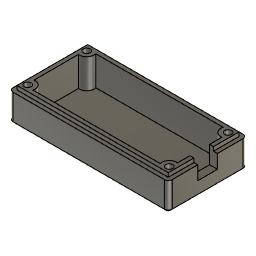
MG996R_Assembly v5 (Autodesk Fusion 360 archive; units mm, degrees)
design "MG996R_Shell_Bottom"
Autodesk Fusion 360 part; units mm, degrees
(part 1 of 2)
sketch "Sketch1" plane through (0, 0, 0) normal (0, 0, 1) x (1, 0, 0)
  line L0 (20.25, 10) -> (-20.25, 10)
  line L1 (-20.25, 10) -> (-20.25, -10)
  line L2 (-20.25, -10) -> (20.25, -10)
  line L3 (20.25, -10) -> (20.25, 10)
  line L4 (20.25, 10) -> (-20.25, -10) construction
  line L5 (-20.25, 10) -> (20.25, -10) construction
  dimension "d1" = 40.5
  dimension "d2" = 20
  constraint horizontal L0
  constraint perpendicular L0 L1
  constraint parallel L0 L2
  constraint parallel L1 L3
  constraint coincident L4 origin
  constraint coincident L5 origin
  measures "d1" distance of L0.start L0.end
  measures "d2" distance of L0.start L2.end
extrude "Extrude1" add sketch "Sketch1" along normal blind 8.53
sketch "Sketch2" plane through (0, 0, 8.53) normal (0, 0, 1) x (-1, 0, 0)
  line L0 (-20.25, 10) -> (-20.25, -10)
  line L1 (-20.25, -10) -> (20.25, -10)
  line L2 (20.25, -10) -> (20.25, 10)
  line L3 (20.25, 10) -> (-20.25, 10)
  line L4 (-18, -7.5) -> (18, -7.5) construction
  line L5 (18, -7.5) -> (18, 7.5) construction
  line L6 (18, 7.5) -> (-18, 7.5) construction
  line L7 (-18, 7.5) -> (-18, -7.5) construction
  line L8 (-18, -7.5) -> (18, 7.5) construction
  line L9 (18, -7.5) -> (-18, 7.5) construction
  circle A0 centre (-18, -7.5) radius 0.875
  circle A1 centre (-18, 7.5) radius 0.875
  circle A2 centre (18, 7.5) radius 0.875
  circle A3 centre (18, -7.5) radius 0.875
  dimension "d6" = 15
  dimension "d7" = 36
  dimension "d8" = 1.75
  constraint horizontal L4
  constraint perpendicular L4 L5
  constraint parallel L4 L6
  constraint parallel L5 L7
  constraint coincident L8 origin
  constraint coincident L9 origin
  constraint coincident L4.start L7.end
  constraint coincident L6.end L7.start
  constraint coincident L5.end L6.start
  constraint coincident L4.end L5.start
  constraint equal A2 A3
  constraint equal A0 A2
  constraint equal A0 A1
  measures "d6" distance of L4.end L5.end
  measures "d7" distance of L4.start L4.end
  measures "d8" diameter of A3
extrude "Extrude2" cut sketch "Sketch2" against normal blind 15 contours A0 | A1 | A2 | A3
sketch "Sketch3" plane through (0, 0, 8.53) normal (0, 0, 1) x (-1, 0, 0)
  circle A0 centre (-18, -7.5) radius 0.875
  circle A1 centre (-18, 7.5) radius 0.875
  circle A2 centre (18, -7.5) radius 0.875
  circle A3 centre (18, 7.5) radius 0.875
  line L0 (-20.25, 10) -> (-20.25, -10)
  line L1 (-20.25, -10) -> (20.25, -10)
  line L2 (20.25, -10) -> (20.25, 10)
  line L3 (20.25, 10) -> (-20.25, 10)
  line L4 (-18.25, -8) -> (18.25, -8)
  line L5 (18.25, -8) -> (18.25, 8)
  line L6 (18.25, 8) -> (-18.25, 8)
  line L7 (-18.25, 8) -> (-18.25, -8)
  line L8 (-18.25, -8) -> (18.25, 8) construction
  line L9 (18.25, -8) -> (-18.25, 8) construction
  circle A4 centre (-18, -7.5) radius 1.875
  circle A5 centre (-18, 7.5) radius 1.875
  circle A6 centre (18, 7.5) radius 1.875
  circle A7 centre (18, -7.5) radius 1.875
  dimension "d11" = 2
  dimension "d13" = 2
  dimension "d14" = 3.75
  constraint horizontal L4
  constraint perpendicular L4 L5
  constraint parallel L4 L6
  constraint parallel L5 L7
  constraint coincident L8 origin
  constraint coincident L9 origin
  constraint concentric A0 A4
  constraint concentric A1 A5
  constraint concentric A3 A6
  constraint concentric A2 A7
  constraint equal A6 A7
  constraint equal A5 A6
  constraint equal A4 A5
  measures "d11" distance of L1 L4
  measures "d13" distance of L0 L7
  measures "d14" diameter of A7
extrude "Extrude3" cut sketch "Sketch3" against normal blind 7.5 contours L4 L5 L6 L7 A4 A5 A6 A7
sketch "Sketch4" plane through (20.25, 0, 0) normal (1, 0, 0) x (0, 1, 0)
  line L0 (-10, 0) -> (10, 0)
  line L1 (10, 0) -> (10, 8.53)
  line L2 (10, 8.53) -> (-10, 8.53)
  line L3 (-10, 8.53) -> (-10, 0)
  line L4 (-2.5, 8.53) -> (2.5, 8.53)
  line L5 (2.5, 8.53) -> (2.5, 4.03)
  line L6 (2.5, 4.03) -> (-2.5, 4.03)
  line L7 (-2.5, 4.03) -> (-2.5, 8.53)
  dimension "d17" = 5
  dimension "d18" = 4.5
  dimension "d19" = 2.5
  constraint horizontal L4
  constraint vertical L5
  constraint horizontal L6
  constraint vertical L7
  constraint coincident L2 L4.start
  measures "d17" distance of L4.start L4.end
  measures "d18" distance of L4.start L6.end
  measures "d19" distance of origin L7
extrude "Extrude4" cut sketch "Sketch4" against normal blind 3 contours L2 L4 L5 L6 L7
sketch "Sketch5" plane through (0, 0, 8.53) normal (0, 0, 1) x (-1, 0, 0)
  line L0 (-20.25, 2.5) -> (-18.25, 2.5)
  line L1 (-18.25, 2.5) -> (-18.25, 5.6417)
  arc A0 (-18.25, 5.6417) -> (-16.1929, 8) centre (-18, 7.5) ccw
  line L2 (-16.1929, 8) -> (16.1929, 8)
  arc A1 (16.1929, 8) -> (18.25, 5.6417) centre (18, 7.5) ccw
  line L3 (18.25, 5.6417) -> (18.25, -5.6417)
  arc A2 (18.25, -5.6417) -> (16.1929, -8) centre (18, -7.5) ccw
  line L4 (16.1929, -8) -> (-16.1929, -8)
  arc A3 (-16.1929, -8) -> (-18.25, -5.6417) centre (-18, -7.5) ccw
  line L5 (-18.25, -5.6417) -> (-18.25, -2.5)
  line L6 (-18.25, -2.5) -> (-20.25, -2.5)
  line L7 (-20.25, -2.5) -> (-20.25, -10)
  line L8 (-20.25, -10) -> (20.25, -10)
  line L9 (20.25, -10) -> (20.25, 10)
  line L10 (20.25, 10) -> (-20.25, 10)
  line L11 (-20.25, 10) -> (-20.25, 2.5)
  circle A4 centre (-18, -7.5) radius 0.875
  circle A5 centre (-18, 7.5) radius 0.875
  circle A6 centre (18, -7.5) radius 0.875
  circle A7 centre (18, 7.5) radius 0.875
  line L12 (19.25, -9) -> (-19.25, -9)
  line L13 (-19.25, -9) -> (-19.25, 9)
  line L14 (-19.25, 9) -> (19.25, 9)
  line L15 (19.25, 9) -> (19.25, -9)
  line L16 (19.25, -9) -> (-19.25, 9) construction
  line L17 (-19.25, -9) -> (19.25, 9) construction
  dimension "d22" = 1
  dimension "d23" = 1
  constraint horizontal L12
  constraint perpendicular L12 L13
  constraint parallel L12 L14
  constraint parallel L13 L15
  constraint coincident L16 origin
  constraint coincident L17 origin
  measures "d22" distance of L8 L12
  measures "d23" distance of L9 L15
extrude "Extrude5" cut sketch "Sketch5" against normal blind 1 contours L0 L6 L7 L8 L9 L10 L11 L12 L13 L14 L15
fillet "Fillet1" radius 1 4 edges at (-20.25, -10, 3.765) (-20.25, 10, 3.765) (20.25, -10, 3.765) (20.25, 10, 3.765)
chamfer "Chamfer1" distance 1 angle 45 8 edges at (0, 10, 0) (-19.9571, 9.7071, 0) (-20.25, 0, 0) (-19.9571, -9.7071, 0) (0, -10, 0) (19.9571, -9.7071, 0) (20.25, 0, 0) (19.9571, 9.7071, 0)
sketch "Sketch6" plane through (0, 0, 0) normal (0, 0, -1) x (1, 0, 0)
  circle A0 centre (-18, 7.5) radius 0.875
  circle A1 centre (-18, -7.5) radius 0.875
  circle A2 centre (18, 7.5) radius 0.875
  circle A3 centre (18, -7.5) radius 0.875
  line L0 (-19.25, -9) -> (19.25, -9)
  line L1 (19.25, -9) -> (19.25, 9)
  line L2 (19.25, 9) -> (-19.25, 9)
  line L3 (-19.25, 9) -> (-19.25, -9)
  circle A4 centre (-19.25, 9) radius 5
  circle A5 centre (19.25, 9) radius 5
  circle A6 centre (19.25, -9) radius 5
  circle A7 centre (-19.25, -9) radius 5
  dimension "d29" = 10
  constraint equal A4 A7
  constraint equal A4 A5
  constraint equal A5 A6
  constraint coincident L2.end L3.start
  constraint coincident L0.start L3.end
  constraint coincident L1.end L2.start
  constraint coincident L0.end L1.start
  measures "d29" diameter of A4
extrude "Extrude6" cut sketch "Sketch6" against normal blind 0.5 contours L0 L3 A7 | L0 L3 A7 | L0 L1 A6 | L0 L1 A6 | L2 L3 A4 | L2 L3 A4 | L1 L2 A5 | L1 L2 A5

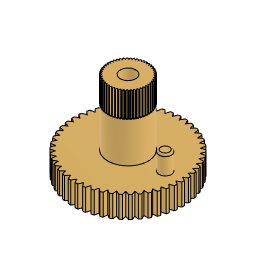
design "MG996R_Gear_4"
Autodesk Fusion 360 part; units mm, degrees
sketch "Sketch1" plane through (0, 0, 0) normal (0, 0, 1) x (1, 0, 0)
  circle A0 centre (0, 0) radius 8.9
  circle A1 centre (0, 0) radius 3.25
  dimension "d1" = 17.8
  dimension "d2" = 6.5
  constraint coincident A0.centre A1.centre
  measures "d1" diameter of A0
  measures "d2" diameter of A1
extrude "Extrude1" add sketch "Sketch1" along normal blind 3.5
sketch "Sketch2" plane through (0, 0, 0) normal (0, 0, -1) x (1, 0, 0)
  circle A0 centre (0, 0) radius 3.25
  circle A1 centre (0, 0) radius 8.9
  circle A2 centre (0, 0) radius 6
  circle A3 centre (0, 0) radius 5
  dimension "d5" = 12
  dimension "d6" = 10
  constraint coincident A0.centre A1.centre
  measures "d5" diameter of A2
  measures "d6" diameter of A3
extrude "Extrude2" add sketch "Sketch2" along normal blind 1 contours A2
extrude "Extrude3" add sketch "Sketch1" along normal blind 14 contours A1
sketch "Sketch4" plane through (0, 0, 14) normal (0, 0, 1) x (-1, 0, 0)
  circle A0 centre (0, 0) radius 3.25
  circle A1 centre (0, 0) radius 1.25
  dimension "d11" = 2.5
  constraint concentric A0 A1
  measures "d11" diameter of A1
extrude "Extrude4" cut sketch "Sketch4" against normal blind 37 contours A1
extrude "Extrude5" cut 1 faces at (3.7314, 0.2484, 0) along direction (0, 0, 1) blind 1.5
sketch "Sketch5" plane through (0, 0, 14) normal (0, 0, 1) x (-1, 0, 0)
  circle A0 centre (0, 0) radius 1.25
  circle A1 centre (0, 0) radius 3.25
  circle A2 centre (0, 0) radius 3.25
  line L0 (0.15, -3.2465) -> (0, -2.9867)
  line L1 (0, -2.9867) -> (-0.15, -3.2465)
  dimension "d16" = 0.3
  dimension "d17" = 0.3
  constraint concentric A0 A2
  constraint coincident A2 L0.start
  constraint coincident A2 L1.end
  constraint equal L0 L1
  constraint equal A1 A2
  constraint vertical A0.centre L0.end
  measures "d16" distance of L0.start L0.end
  measures "d17" distance of L0.start L1.end
extrude "Extrude6" cut sketch "Sketch5" against normal blind 4 contours A1 A2 L0 L1 picked at (0, -3.162)
pattern_circular "C-Pattern1" count 50 over 360 about axis through (0, 0, 14) along (0, 0, -1) of "Extrude6"
sketch "Sketch6" plane through (0, 0, 3.5) normal (0, 0, 1) x (-1, 0, 0)
  circle A0 centre (0, 0) radius 3.25
  circle A1 centre (0, 0) radius 8.9
  circle A2 centre (0, 0) radius 8.9
  line L0 (0.35, -8.8931) -> (0, -8.2869)
  line L1 (0, -8.2869) -> (-0.35, -8.8931)
  dimension "d22" = 0.7
  dimension "d23" = 0.7
  dimension "d24" = 0.7
  constraint coincident A0.centre A1.centre
  constraint coincident A2 L0.start
  constraint coincident A2 L1.end
  constraint equal A1 A2
  constraint vertical A0.centre L0.end
  measures "d22" distance of L0.start L0.end
  measures "d23" distance of L0.end L1.end
  measures "d24" horizontal distance of L0.start L1.end
extrude "Extrude7" cut sketch "Sketch6" against normal blind 6.5 contours A1 A2 L0 L1 picked at (0, -8.6951)
pattern_circular "C-Pattern2" count 50 over 360 about axis through (0, 0, 14) along (0, 0, -1) of "Extrude7"
sketch "Sketch7" plane through (0, 0, 3.5) normal (0, 0, 1) x (-1, 0, 0)
  line L0 (1.0386, -8.2216) -> (1.4618, -8.7791)
  arc A0 (1.4618, -8.7791) -> (1.8726, -8.7008) centre (0, 0) ccw
  line L1 (1.8726, -8.7008) -> (2.0609, -8.0265)
  line L2 (2.0609, -8.0265) -> (2.5506, -8.5267)
  arc A1 (2.5506, -8.5267) -> (2.9484, -8.3975) centre (0, 0) ccw
  line L3 (2.9484, -8.3975) -> (3.0506, -7.705)
  line L4 (3.0506, -7.705) -> (3.5992, -8.1398)
  arc A2 (3.5992, -8.1398) -> (3.9776, -7.9617) centre (0, 0) ccw
  line L5 (3.9776, -7.9617) -> (3.9922, -7.2619)
  line L6 (3.9922, -7.2619) -> (4.591, -7.6245)
  arc A3 (4.591, -7.6245) -> (4.9441, -7.4004) centre (0, 0) ccw
  line L7 (4.9441, -7.4004) -> (4.8709, -6.7042)
  line L8 (4.8709, -6.7042) -> (5.5104, -6.989)
  arc A4 (5.5104, -6.989) -> (5.8326, -6.7224) centre (0, 0) ccw
  line L9 (5.8326, -6.7224) -> (5.6728, -6.0409)
  line L10 (5.6728, -6.0409) -> (6.3429, -6.2432)
  arc A5 (6.3429, -6.2432) -> (6.6292, -5.9384) centre (0, 0) ccw
  line L11 (6.6292, -5.9384) -> (6.3852, -5.2823)
  line L12 (6.3852, -5.2823) -> (7.0754, -5.399)
  arc A6 (7.0754, -5.399) -> (7.3212, -5.0607) centre (0, 0) ccw
  line L13 (7.3212, -5.0607) -> (6.9969, -4.4403)
  line L14 (6.9969, -4.4403) -> (7.6962, -4.4697)
  arc A7 (7.6962, -4.4697) -> (7.8977, -4.1032) centre (0, 0) ccw
  line L15 (7.8977, -4.1032) -> (7.4982, -3.5284)
  line L16 (7.4982, -3.5284) -> (8.1958, -3.4698)
  arc A8 (8.1958, -3.4698) -> (8.3497, -3.081) centre (0, 0) ccw
  line L17 (8.3497, -3.081) -> (7.8813, -2.5608)
  line L18 (7.8813, -2.5608) -> (8.566, -2.4153)
  arc A9 (8.566, -2.4153) -> (8.67, -2.0102) centre (0, 0) ccw
  line L19 (8.67, -2.0102) -> (8.1401, -1.5528)
  line L20 (8.1401, -1.5528) -> (8.8012, -1.3226)
  arc A10 (8.8012, -1.3226) -> (8.8536, -0.9077) centre (0, 0) ccw
  line L21 (8.8536, -0.9077) -> (8.2705, -0.5203)
  line L22 (8.2705, -0.5203) -> (8.8975, -0.2091)
  arc A11 (8.8975, -0.2091) -> (8.8975, 0.2091) centre (0, 0) ccw
  line L23 (8.8975, 0.2091) -> (8.2705, 0.5203)
  line L24 (8.2705, 0.5203) -> (8.8536, 0.9077)
  arc A12 (8.8536, 0.9077) -> (8.8012, 1.3226) centre (0, 0) ccw
  line L25 (8.8012, 1.3226) -> (8.1401, 1.5528)
  line L26 (8.1401, 1.5528) -> (8.67, 2.0102)
  arc A13 (8.67, 2.0102) -> (8.566, 2.4153) centre (0, 0) ccw
  line L27 (8.566, 2.4153) -> (7.8813, 2.5608)
  line L28 (7.8813, 2.5608) -> (8.3497, 3.081)
  arc A14 (8.3497, 3.081) -> (8.1958, 3.4698) centre (0, 0) ccw
  line L29 (8.1958, 3.4698) -> (7.4982, 3.5284)
  line L30 (7.4982, 3.5284) -> (7.8977, 4.1032)
  arc A15 (7.8977, 4.1032) -> (7.6962, 4.4697) centre (0, 0) ccw
  line L31 (7.6962, 4.4697) -> (6.9969, 4.4403)
  line L32 (6.9969, 4.4403) -> (7.3212, 5.0607)
  arc A16 (7.3212, 5.0607) -> (7.0754, 5.399) centre (0, 0) ccw
  line L33 (7.0754, 5.399) -> (6.3852, 5.2823)
  line L34 (6.3852, 5.2823) -> (6.6292, 5.9384)
  arc A17 (6.6292, 5.9384) -> (6.3429, 6.2432) centre (0, 0) ccw
  line L35 (6.3429, 6.2432) -> (5.6728, 6.0409)
  line L36 (5.6728, 6.0409) -> (5.8326, 6.7224)
  arc A18 (5.8326, 6.7224) -> (5.5104, 6.989) centre (0, 0) ccw
  line L37 (5.5104, 6.989) -> (4.8709, 6.7042)
  line L38 (4.8709, 6.7042) -> (4.9441, 7.4004)
  arc A19 (4.9441, 7.4004) -> (4.591, 7.6245) centre (0, 0) ccw
  line L39 (4.591, 7.6245) -> (3.9922, 7.2619)
  line L40 (3.9922, 7.2619) -> (3.9776, 7.9617)
  arc A20 (3.9776, 7.9617) -> (3.5992, 8.1398) centre (0, 0) ccw
  line L41 (3.5992, 8.1398) -> (3.0506, 7.705)
  line L42 (3.0506, 7.705) -> (2.9484, 8.3975)
  arc A21 (2.9484, 8.3975) -> (2.5506, 8.5267) centre (0, 0) ccw
  line L43 (2.5506, 8.5267) -> (2.0609, 8.0265)
  line L44 (2.0609, 8.0265) -> (1.8726, 8.7008)
  arc A22 (1.8726, 8.7008) -> (1.4618, 8.7791) centre (0, 0) ccw
  line L45 (1.4618, 8.7791) -> (1.0386, 8.2216)
  line L46 (1.0386, 8.2216) -> (0.7674, 8.8669)
  arc A23 (0.7674, 8.8669) -> (0.35, 8.8931) centre (0, 0) ccw
  line L47 (0.35, 8.8931) -> (0, 8.2869)
  line L48 (0, 8.2869) -> (-0.35, 8.8931)
  arc A24 (-0.35, 8.8931) -> (-0.7674, 8.8669) centre (0, 0) ccw
  line L49 (-0.7674, 8.8669) -> (-1.0386, 8.2216)
  line L50 (-1.0386, 8.2216) -> (-1.4618, 8.7791)
  arc A25 (-1.4618, 8.7791) -> (-1.8726, 8.7008) centre (0, 0) ccw
  line L51 (-1.8726, 8.7008) -> (-2.0609, 8.0265)
  line L52 (-2.0609, 8.0265) -> (-2.5506, 8.5267)
  arc A26 (-2.5506, 8.5267) -> (-2.9484, 8.3975) centre (0, 0) ccw
  line L53 (-2.9484, 8.3975) -> (-3.0506, 7.705)
  line L54 (-3.0506, 7.705) -> (-3.5992, 8.1398)
  arc A27 (-3.5992, 8.1398) -> (-3.9776, 7.9617) centre (0, 0) ccw
  line L55 (-3.9776, 7.9617) -> (-3.9922, 7.2619)
  line L56 (-3.9922, 7.2619) -> (-4.591, 7.6245)
  arc A28 (-4.591, 7.6245) -> (-4.9441, 7.4004) centre (0, 0) ccw
  line L57 (-4.9441, 7.4004) -> (-4.8709, 6.7042)
  line L58 (-4.8709, 6.7042) -> (-5.5104, 6.989)
  arc A29 (-5.5104, 6.989) -> (-5.8326, 6.7224) centre (0, 0) ccw
  line L59 (-5.8326, 6.7224) -> (-5.6728, 6.0409)
  line L60 (-5.6728, 6.0409) -> (-6.3429, 6.2432)
  arc A30 (-6.3429, 6.2432) -> (-6.6292, 5.9384) centre (0, 0) ccw
  line L61 (-6.6292, 5.9384) -> (-6.3852, 5.2823)
  line L62 (-6.3852, 5.2823) -> (-7.0754, 5.399)
  arc A31 (-7.0754, 5.399) -> (-7.3212, 5.0607) centre (0, 0) ccw
  line L63 (-7.3212, 5.0607) -> (-6.9969, 4.4403)
  line L64 (-6.9969, 4.4403) -> (-7.6962, 4.4697)
  arc A32 (-7.6962, 4.4697) -> (-7.8977, 4.1032) centre (0, 0) ccw
  line L65 (-7.8977, 4.1032) -> (-7.4982, 3.5284)
  line L66 (-7.4982, 3.5284) -> (-8.1958, 3.4698)
  arc A33 (-8.1958, 3.4698) -> (-8.3497, 3.081) centre (0, 0) ccw
  line L67 (-8.3497, 3.081) -> (-7.8813, 2.5608)
  line L68 (-7.8813, 2.5608) -> (-8.566, 2.4153)
  arc A34 (-8.566, 2.4153) -> (-8.67, 2.0102) centre (0, 0) ccw
  line L69 (-8.67, 2.0102) -> (-8.1401, 1.5528)
  line L70 (-8.1401, 1.5528) -> (-8.8012, 1.3226)
  arc A35 (-8.8012, 1.3226) -> (-8.8536, 0.9077) centre (0, 0) ccw
  line L71 (-8.8536, 0.9077) -> (-8.2705, 0.5203)
  line L72 (-8.2705, 0.5203) -> (-8.8975, 0.2091)
  arc A36 (-8.8975, 0.2091) -> (-8.8975, -0.2091) centre (0, 0) ccw
  line L73 (-8.8975, -0.2091) -> (-8.2705, -0.5203)
  line L74 (-8.2705, -0.5203) -> (-8.8536, -0.9077)
  arc A37 (-8.8536, -0.9077) -> (-8.8012, -1.3226) centre (0, 0) ccw
  line L75 (-8.8012, -1.3226) -> (-8.1401, -1.5528)
  line L76 (-8.1401, -1.5528) -> (-8.67, -2.0102)
  arc A38 (-8.67, -2.0102) -> (-8.566, -2.4153) centre (0, 0) ccw
  line L77 (-8.566, -2.4153) -> (-7.8813, -2.5608)
  line L78 (-7.8813, -2.5608) -> (-8.3497, -3.081)
  arc A39 (-8.3497, -3.081) -> (-8.1958, -3.4698) centre (0, 0) ccw
  line L79 (-8.1958, -3.4698) -> (-7.4982, -3.5284)
  line L80 (-7.4982, -3.5284) -> (-7.8977, -4.1032)
  arc A40 (-7.8977, -4.1032) -> (-7.6962, -4.4697) centre (0, 0) ccw
  line L81 (-7.6962, -4.4697) -> (-6.9969, -4.4403)
  line L82 (-6.9969, -4.4403) -> (-7.3212, -5.0607)
  arc A41 (-7.3212, -5.0607) -> (-7.0754, -5.399) centre (0, 0) ccw
  line L83 (-7.0754, -5.399) -> (-6.3852, -5.2823)
  line L84 (-6.3852, -5.2823) -> (-6.6292, -5.9384)
  arc A42 (-6.6292, -5.9384) -> (-6.3429, -6.2432) centre (0, 0) ccw
  line L85 (-6.3429, -6.2432) -> (-5.6728, -6.0409)
  line L86 (-5.6728, -6.0409) -> (-5.8326, -6.7224)
  arc A43 (-5.8326, -6.7224) -> (-5.5104, -6.989) centre (0, 0) ccw
  line L87 (-5.5104, -6.989) -> (-4.8709, -6.7042)
  line L88 (-4.8709, -6.7042) -> (-4.9441, -7.4004)
  arc A44 (-4.9441, -7.4004) -> (-4.591, -7.6245) centre (0, 0) ccw
  line L89 (-4.591, -7.6245) -> (-3.9922, -7.2619)
  line L90 (-3.9922, -7.2619) -> (-3.9776, -7.9617)
  arc A45 (-3.9776, -7.9617) -> (-3.5992, -8.1398) centre (0, 0) ccw
  line L91 (-3.5992, -8.1398) -> (-3.0506, -7.705)
  line L92 (-3.0506, -7.705) -> (-2.9484, -8.3975)
  arc A46 (-2.9484, -8.3975) -> (-2.5506, -8.5267) centre (0, 0) ccw
  line L93 (-2.5506, -8.5267) -> (-2.0609, -8.0265)
  line L94 (-2.0609, -8.0265) -> (-1.8726, -8.7008)
  arc A47 (-1.8726, -8.7008) -> (-1.4618, -8.7791) centre (0, 0) ccw
  line L95 (-1.4618, -8.7791) -> (-1.0386, -8.2216)
  line L96 (-1.0386, -8.2216) -> (-0.7674, -8.8669)
  arc A48 (-0.7674, -8.8669) -> (-0.35, -8.8931) centre (0, 0) ccw
  line L97 (-0.35, -8.8931) -> (0, -8.2869)
  line L98 (0, -8.2869) -> (0.35, -8.8931)
  arc A49 (0.35, -8.8931) -> (0.7674, -8.8669) centre (0, 0) ccw
  line L99 (0.7674, -8.8669) -> (1.0386, -8.2216)
  circle A50 centre (0, 0) radius 3.25
  circle A51 centre (-6, 0) radius 1
  dimension "d29" = 2
  dimension "d30" = 6
  measures "d29" diameter of A51
  measures "d30" distance of A0.centre A51.centre
extrude "Extrude8" add sketch "Sketch7" along normal blind 3 contours A51
fillet "Fillet1" radius 0.3 1 edges at (6.9323, 0.3616, 6.5)
sketch "Sketch8" plane through (0, 0, 1.5) normal (0, 0, -1) x (1, 0, 0)
  circle A0 centre (0, 0) radius 1.25
  circle A1 centre (0, 0) radius 5
  line L0 (-1.5, -1) -> (1.5, -1)
  arc A2 (1.5, -1) -> (1.5, 1) centre (1.5, 0) ccw
  line L1 (1.5, 1) -> (-1.5, 1)
  arc A3 (-1.5, 1) -> (-1.5, -1) centre (-1.5, 0) ccw
  line L2 (-1.5, 0) -> (1.5, 0) construction
  dimension "d35" = 2
  dimension "d36" = 3
  constraint tangent L0 A2
  constraint tangent A2 L1
  constraint parallel L0 L1
  constraint tangent L1 A3
  constraint tangent L0 A3
  constraint horizontal L2
  constraint coincident A0.centre A1.centre
  constraint midpoint L2 A0.centre
  measures "d35" distance of L0 L1
  measures "d36" distance of A3.centre A2.centre
extrude "Extrude9" cut sketch "Sketch8" against normal blind 4 contours A0 L0 A2 L1 | A0 L0 L1 A3

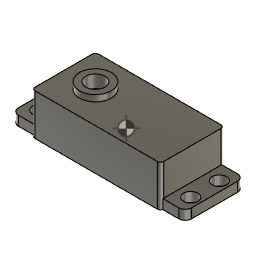
design "MG996R_Shell_Top"
Autodesk Fusion 360 part; units mm, degrees
sketch "Sketch1" plane through (0, 0, 0) normal (0, 0, 1) x (1, 0, 0)
  line L0 (-19.8608, 0) -> (46.1392, 0) construction
  line L1 (-17, -9.25) -> (-10, -9.25)
  line L2 (-10, -9.25) -> (-10, -10)
  line L3 (-10, -10) -> (30.5, -10)
  line L4 (30.5, -10) -> (30.5, -9.25)
  line L5 (30.5, -9.25) -> (37.5, -9.25)
  line L6 (37.5, -9.25) -> (37.5, 0)
  circle A0 centre (-13, -4.5) radius 2.25
  line L7 (-17, -9.25) -> (-17, 0)
  circle A1 centre (34.5, -4.5) radius 2.25
  line L8 (30.5, 10) -> (30.5, 9.25)
  line L9 (-10, 9.25) -> (-10, 10)
  line L10 (-17, 9.25) -> (-17, 0)
  line L11 (37.5, 9.25) -> (37.5, 0)
  line L12 (30.5, 9.25) -> (37.5, 9.25)
  circle A2 centre (-13, 4.5) radius 2.25
  line L13 (-10, 10) -> (30.5, 10)
  line L14 (-17, 9.25) -> (-10, 9.25)
  circle A3 centre (34.5, 4.5) radius 2.25
  point P0 (46.1392, 0)
  point P1 (-19.8608, 0)
  dimension "d1" = 4.5
  dimension "d2" = 10
  dimension "d3" = 4.5
  dimension "d4" = 47.5
  dimension "d5" = 7
  dimension "d6" = 7
  dimension "d7" = 4
  dimension "d8" = 4
  dimension "d9" = 4.5
  dimension "d10" = 4.5
  dimension "d11" = 10
  dimension "d12" = 10
  dimension "d13" = 9.25
  dimension "d14" = 9.25
  constraint horizontal L0
  constraint perpendicular L1 L2
  constraint perpendicular L3 L4
  constraint perpendicular L4 L5
  constraint coincident L0 L6.end
  constraint perpendicular L0 L6
  constraint coincident L0 L7.end
  constraint perpendicular L0 L7
  constraint coincident origin L0
  constraint symmetric P1 L0 L0.start
  constraint symmetric P0 L0 L0.end
  constraint symmetric L0 L1.start L10.start
  constraint symmetric L0 L1.end L9.start
  constraint symmetric L0 L2.end L9.end
  constraint symmetric L0 L3.end L8.start
  constraint symmetric L0 L4.end L8.end
  constraint symmetric L0 L5.end L11.start
  constraint symmetric L0 L6.end L11.end
  constraint symmetric L0 A0 A2
  constraint symmetric L0 L7.end L10.end
  constraint symmetric L0 A1 A3
  measures "d1" diameter of A1
  measures "d2" distance of L0 L3
  measures "d3" distance of L0 A1.centre
  measures "d4" horizontal distance of A0.centre A1.centre
  measures "d5" distance of L2 L7
  measures "d6" distance of L4 L6
  measures "d7" distance of L4 A1.centre
  measures "d8" distance of A0.centre L7
  measures "d9" diameter of A0
  measures "d10" distance of L0 A0.centre
  measures "d11" distance of origin L2
  measures "d12" distance of L0 L3
  measures "d13" distance of L0 L1
  measures "d14" distance of L0 L5
extrude "Extrude1" add sketch "Sketch1" along normal blind 13
sketch "Sketch3" plane through (0, -9.25, 0) normal (0, -1, 0) x (1, 0, 0)
  line L0 (30.5, 0) -> (37.5, 0)
  line L1 (37.5, 0) -> (37.5, 13)
  line L2 (37.5, 13) -> (30.5, 13)
  line L3 (30.5, 13) -> (30.5, 0)
  line L4 (37.5, 0) -> (30.5, 0)
  line L5 (30.5, 0) -> (30.5, 3)
  line L6 (30.5, 3) -> (37.5, 3)
  line L7 (37.5, 3) -> (37.5, 0)
  line L8 (-10, 0) -> (-17, 0)
  line L9 (-17, 0) -> (-17, 3)
  line L10 (-17, 3) -> (-10, 3)
  line L11 (-10, 3) -> (-10, 0)
  dimension "d21" = 3
  dimension "d22" = 3
  constraint horizontal L4
  constraint vertical L5
  constraint horizontal L6
  constraint vertical L7
  constraint coincident L3 L5.end
  constraint coincident L0.end L1.start
  constraint horizontal L8
  constraint vertical L9
  constraint horizontal L10
  constraint vertical L11
  measures "d21" distance of L8.start L10.end
  measures "d22" distance of L0.start L5.end
extrude "Extrude3" cut sketch "Sketch3" against normal blind 26 contours L1 L2 L3 L6
sketch "Sketch4" plane through (0, -9.25, 0) normal (0, -1, 0) x (1, 0, 0)
  line L0 (-17, 0) -> (-10, 0)
  line L1 (-10, 0) -> (-10, 13)
  line L2 (-10, 13) -> (-17, 13)
  line L3 (-17, 13) -> (-17, 0)
  line L4 (-17, 0) -> (-10, 0)
  line L5 (-10, 0) -> (-10, 3)
  line L6 (-10, 3) -> (-17, 3)
  line L7 (-17, 3) -> (-17, 0)
  dimension "d25" = 3
  constraint horizontal L4
  constraint vertical L5
  constraint horizontal L6
  constraint vertical L7
  constraint coincident L1 L5.end
  constraint coincident L0.start L3.end
  measures "d25" distance of L0.start L6.end
extrude "Extrude4" cut sketch "Sketch4" against normal blind 22 contours L1 L2 L3 L6
sketch "Sketch5" plane through (0, 0, 13) normal (0, 0, 1) x (-1, 0, 0)
  line L0 (10, -10) -> (10, 10)
  line L1 (10, 10) -> (-30.5, 10)
  line L2 (-30.5, 10) -> (-30.5, -10)
  line L3 (-30.5, -10) -> (10, -10)
  circle A0 centre (0, 0) radius 3
  dimension "d28" = 6
  constraint coincident A0.centre origin
  measures "d28" diameter of A0
extrude "Extrude5" cut sketch "Sketch5" against normal blind 21 contours A0
sketch "Sketch6" plane through (0, 0, 0) normal (0, 0, -1) x (-1, 0, 0)
  circle A0 centre (0, 0) radius 3
  line L0 (10, -10) -> (10, 10)
  line L1 (10, 10) -> (-33, 10)
  line L2 (-33, 10) -> (-33, -10)
  line L3 (-33, -10) -> (10, -10)
  circle A1 centre (-11, 0) radius 0.75
  circle A2 centre (-20.5, 0) radius 0.75
  circle A3 centre (0, 0) radius 3
  circle A4 centre (-34.5, 4.5) radius 2.25
  circle A5 centre (13, -4.5) radius 2.25
  circle A6 centre (-34.5, -4.5) radius 2.25
  circle A7 centre (13, 4.5) radius 2.25
  line L4 (10, -9.25) -> (17, -9.25)
  line L5 (17, -9.25) -> (17, 9.25)
  line L6 (17, 9.25) -> (10, 9.25)
  line L7 (10, 9.25) -> (10, 10)
  line L8 (10, 10) -> (-30.5, 10)
  line L9 (-30.5, 10) -> (-30.5, 9.25)
  line L10 (-30.5, 9.25) -> (-37.5, 9.25)
  line L11 (-37.5, 9.25) -> (-37.5, -9.25)
  line L12 (-37.5, -9.25) -> (-30.5, -9.25)
  line L13 (-30.5, -9.25) -> (-30.5, -10)
  line L14 (-30.5, -10) -> (10, -10)
  line L15 (10, -10) -> (10, -9.25)
  dimension "d31" = 1.5
  dimension "d32" = 1.5
  dimension "d33" = 11
  dimension "d34" = 9.5
  measures "d31" diameter of A1
  measures "d32" diameter of A2
  measures "d33" distance of A0.centre A1.centre
  measures "d34" distance of A1.centre A2.centre
extrude "Extrude6" cut sketch "Sketch6" against normal blind 12 contours A1 | A2
sketch "Sketch7" plane through (0, 0, 0) normal (0, 0, -1) x (1, 0, 0)
  circle A0 centre (11, 0) radius 0.75
  circle A1 centre (20.5, 0) radius 0.75
  circle A2 centre (0, 0) radius 3
  circle A3 centre (34.5, -4.5) radius 2.25
  circle A4 centre (-13, 4.5) radius 2.25
  circle A5 centre (34.5, 4.5) radius 2.25
  circle A6 centre (-13, -4.5) radius 2.25
  line L0 (-10, 9.25) -> (-17, 9.25)
  line L1 (-17, 9.25) -> (-17, -9.25)
  line L2 (-17, -9.25) -> (-10, -9.25)
  line L3 (-10, -9.25) -> (-10, -10)
  line L4 (-10, -10) -> (30.5, -10)
  line L5 (30.5, -10) -> (30.5, -9.25)
  line L6 (30.5, -9.25) -> (37.5, -9.25)
  line L7 (37.5, -9.25) -> (37.5, 9.25)
  line L8 (37.5, 9.25) -> (30.5, 9.25)
  line L9 (30.5, 9.25) -> (30.5, 10)
  line L10 (30.5, 10) -> (-10, 10)
  line L11 (-10, 10) -> (-10, 9.25)
  line L12 (29.5, 9) -> (-9, 9)
  line L13 (-9, 9) -> (-9, -9)
  line L14 (-9, -9) -> (29.5, -9)
  line L15 (29.5, -9) -> (29.5, 9)
  line L16 (29.5, 9) -> (-9, -9) construction
  line L17 (-9, 9) -> (29.5, -9) construction
  point P0 (10.25, 0)
  dimension "d37" = 1
  dimension "d38" = 1
  dimension "d39" = 1
  dimension "d40" = 1
  constraint horizontal L12
  constraint perpendicular L12 L13
  constraint parallel L12 L14
  constraint parallel L13 L15
  constraint coincident L16 P0
  constraint coincident L17 P0
  measures "d37" distance of L10 L12
  measures "d38" distance of L4 L14
  measures "d39" distance of L5 L15
  measures "d40" distance of L11 L13
extrude "Extrude7" cut sketch "Sketch7" against normal blind 12 contours L12 L13 L14 L15
sketch "Sketch8" plane through (0, 0, 12) normal (0, 0, -1) x (1, 0, 0)
  circle A0 centre (0, 0) radius 3
  line L0 (29.5, -9) -> (29.5, 9)
  line L1 (29.5, 9) -> (-9, 9)
  line L2 (-9, 9) -> (-9, -9)
  line L3 (-9, -9) -> (29.5, -9)
  circle A1 centre (11, 0) radius 0.75
  circle A2 centre (20.5, 0) radius 0.75
  circle A3 centre (11, 0) radius 1.75
  circle A4 centre (20.5, 0) radius 1.75
  dimension "d43" = 1.5
  dimension "d44" = 1.5
  dimension "d45" = 9.5
  dimension "d46" = 11
  dimension "d47" = 3.5
  dimension "d48" = 3.5
  constraint concentric A1 A3
  constraint concentric A2 A4
  measures "d43" diameter of A1
  measures "d44" diameter of A2
  measures "d45" distance of A1.centre A2.centre
  measures "d46" distance of A0.centre A1.centre
  measures "d47" diameter of A3
  measures "d48" diameter of A4
extrude "Extrude8" add sketch "Sketch8" along normal blind 1 contours A3 | A4
sketch "Sketch9" plane through (0, 0, 12) normal (0, 0, -1) x (1, 0, 0)
  circle A0 centre (11, 0) radius 1.75
  circle A1 centre (0, 0) radius 3
  line L0 (29.5, -9) -> (29.5, 9)
  line L1 (29.5, 9) -> (-9, 9)
  line L2 (-9, 9) -> (-9, -9)
  line L3 (-9, -9) -> (29.5, -9)
  circle A2 centre (20.5, 0) radius 1.75
  circle A3 centre (0, 0) radius 3
  circle A4 centre (0, 0) radius 5
  dimension "d51" = 2
  constraint concentric A1 A3
  constraint concentric A3 A4
  measures "d51" distance of A3 A4
extrude "Extrude9" add sketch "Sketch9" along normal blind 1 contours A4
sketch "Sketch10" plane through (0, 0, 13) normal (0, 0, 1) x (-1, 0, 0)
  circle A0 centre (0, 0) radius 3
  line L0 (10, -10) -> (10, 10)
  line L1 (10, 10) -> (-30.5, 10)
  line L2 (-30.5, 10) -> (-30.5, -10)
  line L3 (-30.5, -10) -> (10, -10)
  circle A1 centre (0, 0) radius 3
  circle A2 centre (0, 0) radius 5
  dimension "d54" = 2
  constraint concentric A0 A1
  constraint concentric A1 A2
  measures "d54" distance of A1 A2
extrude "Extrude10" add sketch "Sketch10" along normal blind 2 contours A2
fillet "Fillet1" radius 1 4 edges at (30.5, -10, 6.5) (30.5, 10, 6.5) (-10, -10, 6.5) (-10, 10, 6.5)
fillet "Fillet2" radius 2 4 edges at (37.5, -9.25, 1.5) (37.5, 9.25, 1.5) (-17, -9.25, 1.5) (-17, 9.25, 1.5)
sketch "Sketch11" plane through (0, 0, 12) normal (0, 0, -1) x (1, 0, 0)
  circle A0 centre (0, 0) radius 5 construction
  circle A1 centre (11, 0) radius 1.75 construction
  line L0 (29.5, -9) -> (29.5, 9) construction
  line L1 (29.5, 9) -> (-9, 9) construction
  line L2 (-9, 9) -> (-9, -9) construction
  line L3 (-9, -9) -> (29.5, -9) construction
  circle A2 centre (20.5, 0) radius 1.75 construction
  line L4 (28.25, -7.5) -> (-7.75, -7.5) construction
  line L5 (-7.75, -7.5) -> (-7.75, 7.5) construction
  line L6 (-7.75, 7.5) -> (28.25, 7.5) construction
  line L7 (28.25, 7.5) -> (28.25, -7.5) construction
  circle A3 centre (-7.75, 7.5) radius 0.875
  circle A4 centre (-7.75, -7.5) radius 0.875
  circle A5 centre (28.25, 7.5) radius 0.875
  circle A6 centre (28.25, -7.5) radius 0.875
  circle A7 centre (28.25, 7.5) radius 1.875
  circle A8 centre (28.25, -7.5) radius 1.875
  circle A9 centre (-7.75, -7.5) radius 1.875
  circle A10 centre (-7.75, 7.5) radius 1.875
  line L8 (-9, 10) -> (29.5, 10)
  line L9 (-9, -10) -> (29.5, -10)
  dimension "d63" = 1.25
  dimension "d66" = 1.75
  dimension "d67" = 1
  dimension "d70" = 36
  dimension "d71" = 15
  dimension "d73" = 2.5
  dimension "d74" = 2.5
  dimension "d75" = 1.25
  dimension "d76" = 1.25
  constraint horizontal L4
  constraint vertical L5
  constraint horizontal L6
  constraint vertical L7
  constraint coincident L5.end L6.start
  constraint coincident L4.end L5.start
  constraint coincident L6.end L7.start
  constraint coincident L4.start L7.end
  constraint equal A5 A6
  constraint equal A3 A6
  constraint equal A3 A4
  constraint concentric A6 A8
  constraint concentric A4 A9
  constraint concentric A3 A10
  constraint equal A9 A10
  constraint equal A8 A9
  constraint equal A7 A8
  measures "d63" distance of L2 L5
  measures "d66" diameter of A5
  measures "d67" distance of A5 A7
  measures "d70" distance of L5.end L6.end
  measures "d71" distance of L4.start L6.end
  measures "d73" distance of L6 L8
  measures "d74" distance of L4 L9
  measures "d75" distance of L2 L5
  measures "d76" distance of L0 L7
extrude "Extrude11" add sketch "Sketch11" along normal blind 12
equation "d13 = ( 18.5 / 2 ) * 1 mm"
equation "d14 = ( 18.5 / 2 ) * 1 mm"

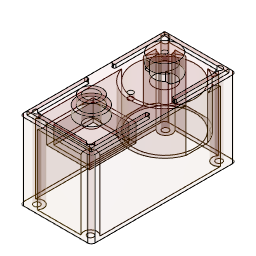
design "MG996R_Shell_Middle"
Autodesk Fusion 360 part; units mm, degrees
sketch "Sketch1" plane through (0, 0, 0) normal (0, 0, 1) x (1, 0, 0)
  line L0 (10, 20.25) -> (-10, 20.25)
  line L1 (-10, 20.25) -> (-10, -20.25)
  line L2 (-10, -20.25) -> (10, -20.25)
  line L3 (10, -20.25) -> (10, 20.25)
  line L4 (10, 20.25) -> (-10, -20.25) construction
  line L5 (-10, 20.25) -> (10, -20.25) construction
  dimension "d1" = 20
  dimension "d2" = 40.5
  constraint horizontal L0
  constraint perpendicular L0 L1
  constraint parallel L0 L2
  constraint parallel L1 L3
  constraint coincident L4 origin
  constraint coincident L5 origin
  measures "d1" distance of L0.start L0.end
  measures "d2" distance of L0.end L1.end
extrude "Extrude1" add sketch "Sketch1" along normal blind 21.5
sketch "Sketch2" plane through (0, 0, 21.5) normal (0, 0, 1) x (-1, 0, 0)
  line L0 (-10, 20.25) -> (-10, -20.25)
  line L1 (-10, -20.25) -> (10, -20.25)
  line L2 (10, -20.25) -> (10, 20.25)
  line L3 (10, 20.25) -> (-10, 20.25)
  line L4 (-8, -18.25) -> (8, -18.25)
  line L5 (8, -18.25) -> (8, 18.25)
  line L6 (8, 18.25) -> (-8, 18.25)
  line L7 (-8, 18.25) -> (-8, -18.25)
  line L8 (-8, -18.25) -> (8, 18.25) construction
  line L9 (8, -18.25) -> (-8, 18.25) construction
  line L10 (-9, -19.25) -> (9, -19.25)
  line L11 (9, -19.25) -> (9, 19.25)
  line L12 (9, 19.25) -> (-9, 19.25)
  line L13 (-9, 19.25) -> (-9, -19.25)
  line L14 (-9, -19.25) -> (9, 19.25) construction
  line L15 (9, -19.25) -> (-9, 19.25) construction
  dimension "d5" = 1
  dimension "d6" = 1
  dimension "d7" = 1
  dimension "d8" = 1
  constraint horizontal L4
  constraint perpendicular L4 L5
  constraint parallel L4 L6
  constraint parallel L5 L7
  constraint coincident L8 origin
  constraint coincident L9 origin
  constraint horizontal L10
  constraint perpendicular L10 L11
  constraint parallel L10 L12
  constraint parallel L11 L13
  constraint coincident L14 origin
  constraint coincident L15 origin
  measures "d5" distance of L4 L10
  measures "d6" distance of L7 L13
  measures "d7" distance of L0 L13
  measures "d8" distance of L1 L10
extrude "Extrude2" add sketch "Sketch2" along normal blind 1 contours L10 L11 L12 L13
sketch "Sketch3" plane through (0, 0, 21.5) normal (0, 0, 1) x (-1, 0, 0)
  line L0 (-8, -18.25) -> (8, -18.25)
  line L1 (8, -18.25) -> (8, 18.25)
  line L2 (8, 18.25) -> (-8, 18.25)
  line L3 (-8, 18.25) -> (-8, -18.25)
  circle A0 centre (0, 10.25) radius 2
  line L4 (10, 20.25) -> (-10, 20.25)
  circle A1 centre (0, -0.75) radius 0.75
  circle A2 centre (0, -10.25) radius 3
  line L5 (-10, -20.25) -> (10, -20.25)
  circle A3 centre (0, -10.25) radius 4
  circle A4 centre (0, 10.25) radius 4
  dimension "d11" = 4
  dimension "d12" = 10
  dimension "d13" = 11
  dimension "d14" = 9.5
  dimension "d16" = 10
  dimension "d17" = 1.5
  dimension "d18" = 6
  dimension "d19" = 8
  dimension "d20" = 8
  constraint vertical A1.centre A2.centre
  constraint vertical A0.centre A1.centre
  constraint vertical origin A1.centre
  constraint concentric A2 A3
  constraint concentric A0 A4
  measures "d11" diameter of A0
  measures "d12" distance of A0.centre L4
  measures "d13" vertical distance of A0.centre A1.centre
  measures "d14" distance of A1.centre A2.centre
  measures "d16" distance of A2.centre L5
  measures "d17" diameter of A1
  measures "d18" diameter of A2
  measures "d19" diameter of A4
  measures "d20" diameter of A3
extrude "Extrude3" add sketch "Sketch3" along normal blind 5 contours A3
extrude "Extrude4" add sketch "Sketch3" along normal blind 5 contours A4
sketch "Sketch4" plane through (0, 0, 26.5) normal (0, 0, 1) x (-1, 0, 0)
  circle A0 centre (0, 10.25) radius 2
  circle A1 centre (0, 10.25) radius 4
  circle A2 centre (0, 10.25) radius 3
  dimension "d25" = 6
  constraint concentric A0 A2
  measures "d25" diameter of A2
extrude "Extrude5" cut sketch "Sketch4" against normal blind 2.5 contours A1
extrude "Extrude6" cut sketch "Sketch3" against normal blind 1.5 contours A1
sketch "Sketch5" plane through (0, 0, 0) normal (0, 0, -1) x (1, 0, 0)
  line L0 (10, -20.25) -> (10, 20.25)
  line L1 (10, 20.25) -> (-10, 20.25)
  line L2 (-10, 20.25) -> (-10, -20.25)
  line L3 (-10, -20.25) -> (10, -20.25)
  line L4 (7.5, 18) -> (-7.5, 18) construction
  line L5 (-7.5, 18) -> (-7.5, -18) construction
  line L6 (-7.5, -18) -> (7.5, -18) construction
  line L7 (7.5, -18) -> (7.5, 18) construction
  line L8 (7.5, 18) -> (-7.5, -18) construction
  line L9 (-7.5, 18) -> (7.5, -18) construction
  circle A0 centre (-7.5, 18) radius 0.875
  circle A1 centre (7.5, 18) radius 0.875
  circle A2 centre (7.5, -18) radius 0.875
  circle A3 centre (-7.5, -18) radius 0.875
  dimension "d30" = 15
  dimension "d31" = 36
  dimension "d32" = 1.75
  constraint horizontal L4
  constraint perpendicular L4 L5
  constraint parallel L4 L6
  constraint parallel L5 L7
  constraint coincident L8 origin
  constraint coincident L9 origin
  constraint coincident L4.end L5.start
  constraint coincident L4.start L7.end
  constraint coincident L6.end L7.start
  constraint coincident L5.end L6.start
  constraint equal A0 A1
  constraint equal A1 A2
  constraint equal A2 A3
  measures "d30" distance of L4.start L4.end
  measures "d31" distance of L4.end L5.end
  measures "d32" diameter of A3
extrude "Extrude7" cut sketch "Sketch5" against normal blind 27 contours A0 | A1 | A2 | A3
sketch "Sketch6" plane through (0, 0, 0) normal (0, 0, -1) x (1, 0, 0)
  circle A0 centre (7.5, 18) radius 0.875
  circle A1 centre (7.5, -18) radius 0.875
  circle A2 centre (-7.5, 18) radius 0.875
  circle A3 centre (-7.5, -18) radius 0.875
  line L0 (10, -20.25) -> (10, 20.25)
  line L1 (10, 20.25) -> (-10, 20.25)
  line L2 (-10, 20.25) -> (-10, -20.25)
  line L3 (-10, -20.25) -> (10, -20.25)
  circle A4 centre (-7.5, 18) radius 1.875
  circle A5 centre (7.5, 18) radius 1.875
  circle A6 centre (7.5, -18) radius 1.875
  circle A7 centre (-7.5, -18) radius 1.875
  line L4 (9, 19.25) -> (-9, 19.25)
  line L5 (-9, 19.25) -> (-9, -19.25)
  line L6 (-9, -19.25) -> (9, -19.25)
  line L7 (9, -19.25) -> (9, 19.25)
  line L8 (9, 19.25) -> (-9, -19.25) construction
  line L9 (-9, 19.25) -> (9, -19.25) construction
  dimension "d35" = 3.75
  dimension "d36" = 1
  dimension "d37" = 1
  constraint concentric A2 A4
  constraint concentric A0 A5
  constraint concentric A1 A6
  constraint concentric A3 A7
  constraint equal A4 A7
  constraint equal A4 A5
  constraint equal A5 A6
  constraint horizontal L4
  constraint perpendicular L4 L5
  constraint parallel L4 L6
  constraint parallel L5 L7
  constraint coincident L8 origin
  constraint coincident L9 origin
  measures "d35" diameter of A7
  measures "d36" distance of L1 L4
  measures "d37" distance of L2 L5
extrude "Extrude8" cut sketch "Sketch6" against normal up to surface (19.5 mm away) contours A4 A5 A6 A7 L4 L5 L6 L7
extrude "Extrude9" cut 1 faces at (0.1483, -10.9, 21.5) along direction (0, 0, -1) blind 15
sketch "Sketch8" plane through (0, 0, 26.5) normal (0, 0, 1) x (-1, 0, 0)
  circle A0 centre (0, -10.25) radius 3
  circle A1 centre (0, -10.25) radius 4
  circle A2 centre (0, -10.25) radius 4
  constraint concentric A0 A2
extrude "Extrude10" add sketch "Sketch8" against normal blind 2.5 contours A0
ref_plane "WorkPlane1" through (0, 6.25, 22) normal (0, -1, 0) x (1, 0, 0)
sketch "Sketch10" plane through (0, 6.25, 22) normal (0, -1, 0) x (1, 0, 0)
  line L0 (-4, 2) -> (4, 2)
  line L1 (4, 2) -> (4, -0.5)
  line L2 (4, -0.5) -> (-4, -0.5)
  line L3 (-4, -0.5) -> (-4, 2)
  constraint horizontal L0
  constraint vertical L1
  constraint horizontal L2
  constraint vertical L3
extrude "Extrude11" cut sketch "Sketch10" against normal blind 2
sketch "Sketch11" plane through (0, 0, 26.5) normal (0, 0, 1) x (-1, 0, 0)
  circle A0 centre (0, -10.25) radius 4
  circle A1 centre (0, -10.25) radius 0.75
  dimension "d47" = 1.5
  constraint concentric A0 A1
  measures "d47" diameter of A1
extrude "Extrude12" cut sketch "Sketch11" against normal blind 1.5 contours A1
sketch "Sketch12" plane through (0, 0, 21.5) normal (0, 0, 1) x (-1, 0, 0)
  arc A0 (-3.4641, -8.25) -> (3.4641, -8.25) centre (0, -10.25) ccw
  line L0 (-3.4641, -8.25) -> (-2.2361, -8.25)
  arc A1 (-2.2361, -8.25) -> (2.2361, -8.25) centre (0, -10.25) ccw
  line L1 (2.2361, -8.25) -> (3.4641, -8.25)
  arc A2 (-8, 17.2819) -> (-6.6615, 18.25) centre (-7.5, 18) ccw
  line L2 (-8, 17.2819) -> (-8, -17.2819)
  arc A3 (-6.6615, -18.25) -> (-8, -17.2819) centre (-7.5, -18) ccw
  line L3 (-6.6615, -18.25) -> (6.6615, -18.25)
  arc A4 (8, -17.2819) -> (6.6615, -18.25) centre (7.5, -18) ccw
  line L4 (8, -17.2819) -> (8, 17.2819)
  arc A5 (6.6615, 18.25) -> (8, 17.2819) centre (7.5, 18) ccw
  line L5 (6.6615, 18.25) -> (-6.6615, 18.25)
  circle A6 centre (0, -0.75) radius 0.75
  circle A7 centre (0, 10.25) radius 4
  circle A8 centre (0, -10.25) radius 3
  dimension "d50" = 6
  constraint concentric A0 A8
  measures "d50" diameter of A8
extrude "Extrude13" cut sketch "Sketch12" against normal blind 4 contours A1 A8
sketch "Sketch13" plane through (0, 0, 21.5) normal (0, 0, 1) x (-1, 0, 0)
  arc A0 (2.2361, -8.25) -> (-2.2361, -8.25) centre (0, -10.25) ccw
  line L0 (2.2361, -8.25) -> (3.4641, -8.25)
  arc A1 (-3.4641, -8.25) -> (3.4641, -8.25) centre (0, -10.25) ccw
  line L1 (-3.4641, -8.25) -> (-2.2361, -8.25)
  arc A2 (-8, 17.2819) -> (-6.6615, 18.25) centre (-7.5, 18) ccw
  line L2 (-8, 17.2819) -> (-8, -17.2819)
  arc A3 (-6.6615, -18.25) -> (-8, -17.2819) centre (-7.5, -18) ccw
  line L3 (-6.6615, -18.25) -> (6.6615, -18.25)
  arc A4 (8, -17.2819) -> (6.6615, -18.25) centre (7.5, -18) ccw
  line L4 (8, -17.2819) -> (8, 17.2819)
  arc A5 (6.6615, 18.25) -> (8, 17.2819) centre (7.5, 18) ccw
  line L5 (6.6615, 18.25) -> (-6.6615, 18.25)
  circle A6 centre (0, -0.75) radius 0.75
  circle A7 centre (0, 10.25) radius 4
  line L6 (-12.9231, -4.25) -> (12.9231, -4.25)
  line L7 (12.9231, -4.25) -> (12.9231, 2.75)
  line L8 (12.9231, 2.75) -> (-12.9231, 2.75)
  line L9 (-12.9231, 2.75) -> (-12.9231, -4.25)
  line L10 (-12.9231, -4.25) -> (12.9231, 2.75) construction
  line L11 (12.9231, -4.25) -> (-12.9231, 2.75) construction
  point P0 (0, -0.75)
  dimension "d53" = 7
  constraint horizontal L6
  constraint perpendicular L6 L7
  constraint parallel L6 L8
  constraint parallel L7 L9
  constraint coincident L10 P0
  constraint coincident L11 P0
  constraint coincident P0 A6.centre
  measures "d53" distance of L6.end L7.end
extrude "Extrude14" cut sketch "Sketch13" along normal blind 3 contours L2 L6 L8 L9 | L4 L6 L7 L8
fillet "Fillet1" radius 0.35 8 edges at (-9, 4.25, 22) (-8, 4.25, 22) (-9, -2.75, 22) (-8, -2.75, 22) (8, 4.25, 22) (9, 4.25, 22) (8, -2.75, 22) (9, -2.75, 22)
fillet "Fillet2" radius 1 4 edges at (-10, -20.25, 10.75) (10, -20.25, 10.75) (-10, 20.25, 10.75) (10, 20.25, 10.75)
sketch "Sketch14" plane through (0, 0, 19.5) normal (0, 0, -1) x (1, 0, 0)
  circle A0 centre (0, -10.25) radius 3
  circle A1 centre (0, 10.25) radius 2
  arc A2 (-6.1025, -19.25) -> (-9, -16.875) centre (-7.5, -18) ccw
  line L0 (-6.1025, -19.25) -> (6.1025, -19.25)
  arc A3 (9, -16.875) -> (6.1025, -19.25) centre (7.5, -18) ccw
  line L1 (9, -16.875) -> (9, 16.875)
  arc A4 (6.1025, 19.25) -> (9, 16.875) centre (7.5, 18) ccw
  line L2 (6.1025, 19.25) -> (-6.1025, 19.25)
  arc A5 (-9, 16.875) -> (-6.1025, 19.25) centre (-7.5, 18) ccw
  line L3 (-9, 16.875) -> (-9, -16.875)
  circle A6 centre (0, -10.25) radius 8.5
  circle A7 centre (0, -10.25) radius 9.5
  dimension "d60" = 17
  dimension "d61" = 1
  constraint concentric A0 A6
  constraint concentric A6 A7
  measures "d60" diameter of A6
  measures "d61" distance of A6 A7
extrude "Extrude15" add sketch "Sketch14" along normal blind 12 contours A2 L0 A3 L1 L3 A7
sketch "Sketch15" plane through (0, 0, 19.5) normal (0, 0, -1) x (1, 0, 0)
  circle A0 centre (0, 10.25) radius 2
  arc A1 (9, -7.2086) -> (-9, -7.2086) centre (0, -10.25) ccw
  line L0 (9, -7.2086) -> (9, 16.875)
  arc A2 (6.1025, 19.25) -> (9, 16.875) centre (7.5, 18) ccw
  line L1 (6.1025, 19.25) -> (-6.1025, 19.25)
  arc A3 (-9, 16.875) -> (-6.1025, 19.25) centre (-7.5, 18) ccw
  line L2 (-9, 16.875) -> (-9, -7.2086)
  line L3 (5, 15.75) -> (-5, 15.75)
  line L4 (-5, 15.75) -> (-5, 4.75)
  line L5 (-5, 4.75) -> (5, 4.75)
  line L6 (5, 4.75) -> (5, 15.75)
  line L7 (5, 15.75) -> (-5, 4.75) construction
  line L8 (-5, 15.75) -> (5, 4.75) construction
  line L9 (6, 16.75) -> (-6, 16.75)
  line L10 (-6, 16.75) -> (-6, 3.75)
  line L11 (-6, 3.75) -> (6, 3.75)
  line L12 (6, 3.75) -> (6, 16.75)
  line L13 (6, 16.75) -> (-6, 3.75) construction
  line L14 (-6, 16.75) -> (6, 3.75) construction
  point P0 (0, 10.25)
  point P1 (0, 10.25)
  dimension "d64" = 10
  dimension "d65" = 11
  dimension "d66" = 1
  dimension "d67" = 1
  constraint horizontal L3
  constraint perpendicular L3 L4
  constraint parallel L3 L5
  constraint parallel L4 L6
  constraint coincident L7 P1
  constraint coincident L8 P1
  constraint coincident P0 A0.centre
  constraint horizontal L9
  constraint perpendicular L9 L10
  constraint parallel L9 L11
  constraint parallel L10 L12
  constraint coincident L13 P1
  constraint coincident L14 P1
  constraint coincident P1 P0
  measures "d64" distance of L3.start L3.end
  measures "d65" distance of L3.start L5.end
  measures "d66" distance of L6 L12
  measures "d67" distance of L3 L9
extrude "Extrude16" add sketch "Sketch15" along normal blind 5 contours L9 L10 L11 L12
equation "d35 = 1.75 mm + 2 mm"

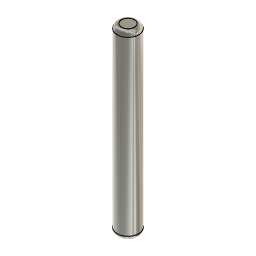
design "MG996R_Pin_Long"
Autodesk Fusion 360 part; units mm, degrees
sketch "Sketch1" plane through (0, 0, 0) normal (0, 0, 1) x (1, 0, 0)
  circle A0 centre (0, 0) radius 0.75
  dimension "d1" = 1.5
  constraint coincident A0.centre origin
  measures "d1" diameter of A0
extrude "Extrude1" add sketch "Sketch1" along normal blind 12.5
fillet "Fillet1" radius 0.3 2 edges at (-0.6992, -0.2712, 12.5) (-0.6992, -0.2712, 0)

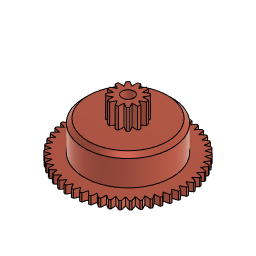
design "MG996R_Gear_2"
Autodesk Fusion 360 part; units mm, degrees
sketch "Sketch1" plane through (0, 0, 0) normal (0, 0, 1) x (1, 0, 0)
  circle A0 centre (0, 0) radius 7.5
  circle A1 centre (0, 0) radius 5.5
  circle A2 centre (0, 0) radius 2
  dimension "d1" = 15
  dimension "d2" = 11
  dimension "d3" = 4
  constraint coincident A0.centre A1.centre
  measures "d1" diameter of A0
  measures "d2" diameter of A1
  measures "d3" diameter of A2
extrude "Extrude1" add sketch "Sketch1" along normal blind 7.3 contours A2 makes body 1
extrude "Extrude2" add sketch "Sketch1" along normal blind 1 separate body contours A0 makes body 2
extrude "Extrude3" add sketch "Sketch1" along normal blind 4.7 contours A1 bodies 1 2
sketch "Sketch2" plane through (0, 0, 0) normal (0, 0, -1) x (1, 0, 0)
  circle A0 centre (0, 0) radius 7.5
  circle A1 centre (0, 0) radius 4.25
  dimension "d10" = 8.5
  constraint concentric A0 A1
  measures "d10" diameter of A1
extrude "Extrude4" cut sketch "Sketch2" against normal blind 3.5 contours A1 bodies 1
sketch "Sketch3" plane through (0, 0, 7.3) normal (0, 0, 1) x (-1, 0, 0)
  circle A0 centre (0, 0) radius 2
  circle A1 centre (0, 0) radius 0.75
  dimension "d13" = 1.5
  constraint concentric A0 A1
  measures "d13" diameter of A1
extrude "Extrude5" cut sketch "Sketch3" against normal blind 24 contours A1 bodies 1
chamfer "Chamfer1" distance 0.5 angle 45 1 edges at (-5.1278, -1.9889, 4.7) on bodies 1
sketch "Sketch4" plane through (0, 0, 7.3) normal (0, 0, 1) x (-1, 0, 0)
  circle A0 centre (0, 0) radius 0.75
  circle A1 centre (0, 0) radius 2
  circle A2 centre (0, 0) radius 2
  line L0 (0.35, -1.9691) -> (0, -1.3629)
  line L1 (0, -1.3629) -> (-0.35, -1.9691)
  dimension "d17" = 0.7
  dimension "d18" = 0.7
  constraint concentric A0 A2
  constraint coincident A2 L0.start
  constraint coincident A2 L1.end
  constraint equal L0 L1
  constraint vertical A0.centre L0.end
  constraint equal A1 A2
  measures "d17" distance of L0.start L0.end
  measures "d18" horizontal distance of L0.start L1.end
extrude "Extrude6" cut sketch "Sketch4" against normal blind 2.6 contours A1 A2 L0 L1 picked at (0, -1.7853) bodies 1
pattern_circular "C-Pattern1" count 12 over 360 about axis through (0, 0, 7.3) along (0, 0, -1) of "Extrude6"
sketch "Sketch5" plane through (0, 0, 1) normal (0, 0, 1) x (-1, 0, 0)
  circle A0 centre (0, 0) radius 5.5
  circle A1 centre (0, 0) radius 7.5
  circle A2 centre (0, 0) radius 7.5
  line L0 (0.35, -7.4918) -> (0, -6.8856)
  line L1 (0, -6.8856) -> (-0.35, -7.4918)
  dimension "d25" = 0.7
  dimension "d26" = 0.7
  constraint coincident A0.centre A1.centre
  constraint equal A1 A2
  constraint coincident A2 L0.start
  constraint coincident A2 L1.end
  constraint equal L0 L1
  constraint vertical A0.centre L0.end
  measures "d25" horizontal distance of L0.start L1.end
  measures "d26" distance of L0.start L0.end
extrude "Extrude7" cut sketch "Sketch5" against normal blind 3.5 contours A1 A2 L0 L1 picked at (0, -7.2946) bodies 1
pattern_circular "C-Pattern2" count 50 over 360 about axis through (0, 0, 7.3) along (0, 0, -1) of "Extrude7"
chamfer "Chamfer2" distance 0.5 angle 45 2 edges at (-3.9624, -1.5369, 3.5) (-3.9624, -1.5369, 0) on bodies 1

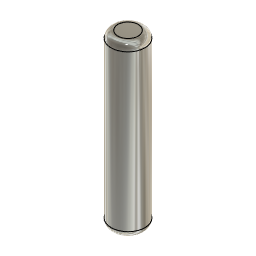
design "MG996R_Pin_Short"
Autodesk Fusion 360 part; units mm, degrees
sketch "Sketch1" plane through (0, 0, 0) normal (0, 0, 1) x (1, 0, 0)
  circle A0 centre (0, 0) radius 0.75
  dimension "d1" = 1.5
  constraint coincident A0.centre origin
  measures "d1" diameter of A0
extrude "Extrude1" add sketch "Sketch1" along normal blind 7.5
fillet "Fillet1" radius 0.3 2 edges at (-0.6992, -0.2712, 7.5) (-0.6992, -0.2712, 0)

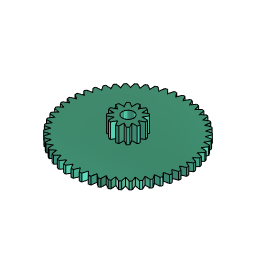
design "MG996R_Gear_1"
Autodesk Fusion 360 part; units mm, degrees